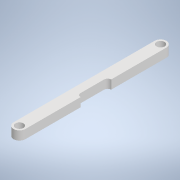
# Autodesk Inventor part: MainLink
Saved by Autodesk Inventor 2022.6 (Build 266554000, 554)
## iProperties
Created: 2024-10-23
Part Number: MainLink
Material: Generic
Document SubType Name: Modeling
Designer: Zhong
Density: 1 g/cm^3
Appearance: Default
Author: Zhong
Autodesk Inventor part; units mm, degrees
ref_plane "YZ Plane" through (0, 0, 0) normal (1, 0, 0) x (0, 1, 0)
ref_plane "XZ Plane" through (0, 0, 0) normal (0, 1, 0) x (-1, 0, 0)
ref_plane "XY Plane" through (0, 0, 0) normal (0, 0, 1) x (1, 0, 0)
sketch "Sketch1" plane through (0, 0, 0) normal (0, 1, 0) x (-1, 0, 0)
  line L0 (0, 30) -> (0, -30) construction
  line L1 (-2.5, 30) -> (-2.5, -30)
  line L2 (2.5, -30) -> (2.5, 30)
  arc A0 (2.5, 30) -> (-2.5, 30) centre (0, 30) ccw
  arc A1 (-2.5, -30) -> (2.5, -30) centre (0, -30) ccw
  point P0 (0, 0)
  point P1 (0, 0)
  dimension "d0" = 60
  dimension "d1" = 5
  constraints: 8 end point, 4 point on circle, 4 tangent, 2 centre point, 1 coincident, 1 midpoint, 1 parallel, 1 vertical
  measures "d0" distance of L0.start L0.end
  measures "d1" diameter of A1
extrude "Extrusion1" add sketch "Sketch1" along normal blind 3.75
sketch "Sketch2" plane through (0, 3.75, 0) normal (0, 1, 0) x (1, 0, 0)
  arc A0 (2.5, 30) -> (-2.5, 30) centre (0, 30) ccw projected
  line L0 (-2.5, 30) -> (-2.5, -30) projected
  arc A1 (-2.5, -30) -> (2.5, -30) centre (0, -30) ccw projected
  line L1 (2.5, -30) -> (2.5, 30) projected
  point P0 (0, 0)
  constraints: 2 coincident
hole "Hole1" at (0, 3.75, 30) at (0, 3.75, -30) direction (0, -1, 0) diameter 3.4 end through all
sketch "Sketch3" plane through (0, 3.75, 0) normal (0, 1, 0) x (1, 0, 0)
  line L0 (2.5, 5) -> (2.5, -5) construction
  line L1 (2.5, -30) -> (2.5, 30) projected
  line L2 (1, 5) -> (1, -5)
  line L3 (4, -5) -> (4, 5)
  arc A0 (4, 5) -> (1, 5) centre (2.5, 5) ccw
  arc A1 (1, -5) -> (4, -5) centre (2.5, -5) ccw
  point P0 (0, 0)
  point P1 (2.5, 0)
  point P2 (2.5, -6.5)
  point P3 (2.5, 6.5)
  dimension "d11" = 5
  dimension "d12" = 3
  constraints: 8 end point, 4 point on circle, 4 tangent, 2 centre point, 2 midpoint, 1 parallel, 1 point on line
  measures "d11" distance of point (2.5, 0) L0.end
  measures "d12" diameter of A1
extrude "Extrusion2" cut sketch "Sketch3" against normal through all contours A1 L2 A0 L1
body "Solid1"
